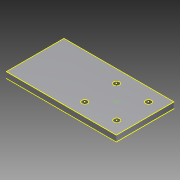
# Autodesk Inventor part: Part4
Saved by Autodesk Inventor 2012 (Build 160160000, 160)
## iProperties
Created: 2012-06-20
Part Number: Part4
Material: Default
Document SubType Name: Modeling
Designer: wberry
Density: 1 g/cm^3
Author: wberry
Autodesk Inventor part; units mm, degrees
ref_plane "YZ Plane" through (0, 0, 0) normal (1, 0, 0) x (0, 1, 0)
ref_plane "XZ Plane" through (0, 0, 0) normal (0, 1, 0) x (-1, 0, 0)
ref_plane "XY Plane" through (0, 0, 0) normal (0, 0, 1) x (1, 0, 0)
sketch "Sketch1" plane through (0, 0, 0) normal (0, 0, 1) x (1, 0, 0)
  line L0 (0, 0) -> (120.5, 0)
  line L1 (120.5, 0) -> (120.5, 63.11)
  line L2 (120.5, 63.11) -> (0, 63.11)
  line L3 (0, 63.11) -> (0, 0)
  dimension "d0" = 120.5
  dimension "d1" = 63.11
  constraints: 8 end point, 2 parallel, 1 horizontal, 1 perpendicular
  measures "d0" distance of L2.end L1.end
  measures "d1" distance of L1.end L0.end
extrude "Extrusion2" add sketch "Sketch1" along normal blind 6.45
sketch "Sketch2" plane through (0, 0, 6.45) normal (0, 0, 1) x (1, 0, 0)
  point P0 (71.68, 14.22)
  point P1 (106.68, 14.22)
  point P2 (106.68, 49.08)
  point P3 (71.68, 49.08)
hole "Hole1" at (71.68, 14.22, 6.45) at (106.68, 14.22, 6.45) at (106.68, 49.08, 6.45) at (71.68, 49.08, 6.45) direction (0, 0, -1) diameter 6.35 end through all
sketch "Sketch3" plane through (0, 0, 6.45) normal (0, 0, 1) x (1, 0, 0)
  circle A0 centre (71.68, 49.08) radius 3.175 projected
  circle A1 centre (106.68, 49.08) radius 3.175 projected
  circle A2 centre (106.68, 14.22) radius 3.175 projected
  circle A3 centre (71.68, 14.22) radius 3.175 projected
  line L0 (0, 0) -> (0, 63.11) projected
  line L1 (120.5, 0) -> (0, 0) projected
  line L2 (120.5, 63.11) -> (120.5, 0) projected
  line L3 (0, 63.11) -> (120.5, 63.11) projected
sketch "Sketch4" plane through (0, 0, 0) normal (0, 0, -1) x (-1, 0, 0)
  circle A0 centre (-71.68, 49.08) radius 3.175 projected
  circle A1 centre (-106.68, 49.08) radius 3.175 projected
  circle A2 centre (-106.68, 14.22) radius 3.175 projected
  circle A3 centre (-71.68, 14.22) radius 3.175 projected
  line L0 (0, 0) -> (-120.5, 0) projected
  line L1 (0, 63.11) -> (0, 0) projected
  line L2 (-120.5, 63.11) -> (0, 63.11) projected
  line L3 (-120.5, 0) -> (-120.5, 63.11) projected
  point P0 (-89.18, 31.555)
sketch "Sketch5" plane through (0, 0, 0) normal (0, 0, -1) x (-1, 0, 0)
  circle A0 centre (-71.68, 49.08) radius 3.175 projected
  circle A1 centre (-106.68, 49.08) radius 3.175 projected
  circle A2 centre (-106.68, 14.22) radius 3.175 projected
  circle A3 centre (-71.68, 14.22) radius 3.175 projected
  line L0 (0, 0) -> (-120.5, 0) projected
  line L1 (0, 63.11) -> (0, 0) projected
  line L2 (-120.5, 63.11) -> (0, 63.11) projected
  line L3 (-120.5, 0) -> (-120.5, 63.11) projected
sketch "Sketch6" plane through (0, 0, 6.45) normal (0, 0, 1) x (1, 0, 0)
  circle A0 centre (71.68, 49.08) radius 3.175 projected
  circle A1 centre (106.68, 49.08) radius 3.175 projected
  circle A2 centre (106.68, 14.22) radius 3.175 projected
  circle A3 centre (71.68, 14.22) radius 3.175 projected
  line L0 (0, 0) -> (0, 63.11) projected
  line L1 (120.5, 0) -> (0, 0) projected
  line L2 (120.5, 63.11) -> (120.5, 0) projected
  line L3 (0, 63.11) -> (120.5, 63.11) projected
  point P0 (89.18, 31.555)
body "Solid2"
